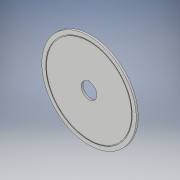
# Autodesk Inventor part: PlateCenter
Saved by Autodesk Inventor 2019 (Build 230136000, 136)
## iProperties
Created: 2019-04-16
Part Number: PlateCenter
Material: Generic
Document SubType Name: Modeling
Designer: samson.bailor
Density: 1 g/cm^3
Appearance: Default
Author: samson.bailor
Autodesk Inventor part; units mm, degrees
ref_plane "YZ Plane" through (0, 0, 0) normal (1, 0, 0) x (0, 1, 0)
ref_plane "XZ Plane" through (0, 0, 0) normal (0, 1, 0) x (-1, 0, 0)
ref_plane "XY Plane" through (0, 0, 0) normal (0, 0, 1) x (1, 0, 0)
sketch "Sketch1" plane through (0, 0, 0) normal (0, 0, 1) x (1, 0, 0)
  circle A0 centre (0, 0) radius 152.4
  circle A1 centre (0, 0) radius 23.8125
  dimension "d0" = 304.8
  dimension "d2" = 47.625
  constraints: 2 centre point, 1 coincident
  measures "d0" diameter of A0
  measures "d2" diameter of A1
extrude "Extrusion1" add sketch "Sketch1" along normal blind 6.35
sketch "Sketch2" plane through (0, 0, 6.35) normal (0, 0, 1) x (1, 0, 0)
  circle A0 centre (0, 0) radius 23.8125 projected
  circle A1 centre (0, 0) radius 139.7
  circle A2 centre (0, 0) radius 137.16
  dimension "d5" = 279.4
  dimension "d6" = 274.32
  constraints: 2 centre point, 2 coincident
  measures "d5" diameter of A1
  measures "d6" diameter of A2
extrude "Extrusion2" cut sketch "Sketch2" against normal blind 1.27 contours A1
sketch "Sketch3" plane through (0, 0, 0) normal (0, 0, -1) x (-1, 0, 0)
  circle A0 centre (0, 0) radius 137.16
  circle A1 centre (0, 0) radius 140.2489
  constraints: 2 centre point, 2 coincident
extrude "Extrusion3" cut sketch "Sketch3" against normal blind 1.27
sketch "Sketch4" plane through (0, 0, 6.35) normal (0, 0, 1) x (1, 0, 0)
  arc A0 (-2.54, 25.2727) -> (2.54, 25.2727) centre (0, 0) ccw
  line L0 (0, 26.67) -> (2.54, 26.67)
  line L1 (0, 26.67) -> (-2.54, 26.67)
  line L2 (-2.54, 26.67) -> (-2.54, 25.2727)
  line L3 (2.54, 26.67) -> (2.54, 25.2727)
  dimension "d11" = 50.8
  dimension "d13" = 2.54
  dimension "d14" = 2.54
  constraints: 8 end point, 2 horizontal, 2 point on circle, 2 vertical, 1 centre point, 1 coincident
  measures "d11" diameter of A0
  measures "d13" distance of L0.start L0.end
  measures "d14" distance of L0.start L1.end
extrude "Extrusion4" cut sketch "Sketch4" against normal blind 25.4
body "Solid1"
